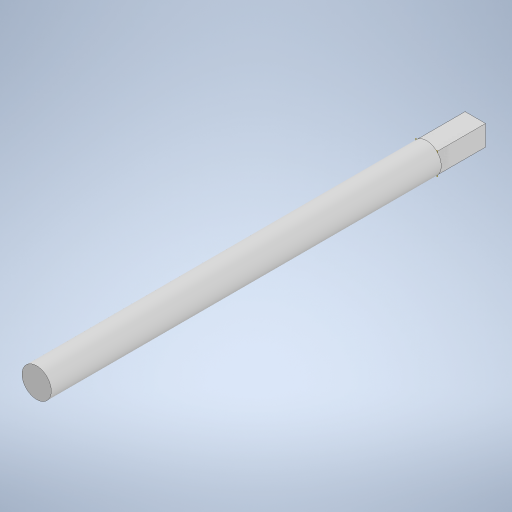
# Autodesk Inventor part: Pieza1
Saved by Autodesk Inventor 2023 (Build 270158000, 158)
## iProperties
Created: 2023-06-06
Part Number: Pieza1
Material: Genérico
Document SubType Name: Modeling
Designer: sergi
Density: 1 g/cm^3
Appearance: Valor por defecto
Author: sergi
Autodesk Inventor part; units mm, degrees
ref_plane "YZ Plane" through (0, 0, 0) normal (1, 0, 0) x (0, 1, 0)
ref_plane "XZ Plane" through (0, 0, 0) normal (0, 1, 0) x (-1, 0, 0)
ref_plane "XY Plane" through (0, 0, 0) normal (0, 0, 1) x (1, 0, 0)
sketch "Boceto1" plane through (0, 0, 0) normal (0, 0, 1) x (1, 0, 0)
  line L0 (3.15, -3.15) -> (-3.15, -3.15)
  line L1 (-3.15, -3.15) -> (-3.15, 3.15)
  line L2 (-3.15, 3.15) -> (3.15, 3.15)
  line L3 (3.15, 3.15) -> (3.15, -3.15)
  line L4 (3.15, -3.15) -> (-3.15, 3.15) construction
  line L5 (-3.15, -3.15) -> (3.15, 3.15) construction
  point P0 (0, 0)
  dimension "d0" = 6.3
  dimension "d1" = 6.3
  constraints: 12 end point, 2 midpoint, 2 parallel, 1 horizontal, 1 perpendicular
  measures "d0" distance of L1.end L2.end
  measures "d1" distance of L0.end L1.end
extrude "Extrusión1" add sketch "Boceto1" along normal blind 135
ref_plane "Plano de trabajo2" through (0, 0, 15) normal (0, 0, -1) x (-1, 0, 0)
sketch "Boceto3" plane through (0, 0, 15) normal (0, 0, -1) x (-1, 0, 0)
  circle A0 centre (0, 0) radius 4.5
  dimension "d9" = 9
  constraints: 1 centre point, 1 coincident
  measures "d9" diameter of A0
extrude "Extrusión3" add sketch "Boceto3" against normal up to surface (120 mm away)
